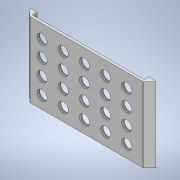
# Autodesk Inventor part: PalmSupport
Saved by Autodesk Inventor 2020 (Build 240168000, 168)
## iProperties
Created: 2019-10-21
Part Number: PalmSupport
Material: Generic
Document SubType Name: Modeling
Designer: ayad493
Density: 1 g/cm^3
Appearance: Default
Author: ayad493
Autodesk Inventor part; units mm, degrees
ref_plane "YZ Plane" through (0, 0, 0) normal (1, 0, 0) x (0, 1, 0)
ref_plane "XZ Plane" through (0, 0, 0) normal (0, 1, 0) x (-1, 0, 0)
ref_plane "XY Plane" through (0, 0, 0) normal (0, 0, 1) x (1, 0, 0)
sketch "Sketch1" plane through (0, 0, 0) normal (0, 0, 1) x (1, 0, 0)
  line L0 (0, 0) -> (51.5, 0)
  line L1 (51.5, 0) -> (51.5, 30)
  line L2 (51.5, 30) -> (0, 30)
  line L3 (0, 30) -> (0, 0)
  dimension "d0" = 51.5
  dimension "d1" = 30
  constraints: 8 end point, 2 parallel, 1 horizontal, 1 perpendicular
  measures "d0" distance of L2.end L1.end
  measures "d1" distance of L1.end L0.end
extrude "Extrusion1" add sketch "Sketch1" along normal blind 2.9
sketch "Sketch2" plane through (0, 0, 0) normal (0, -1, 0) x (1, 0, 0)
  line L0 (0, 0) -> (0, 2.9) projected
  line L1 (0, 2.9) -> (3, 2.9)
  line L2 (51.5, 2.9) -> (0, 2.9) projected
  line L3 (51.5, 0) -> (0, 0) projected
  line L4 (3, 2.9) -> (0, 0)
  line L5 (51.5, 2.9) -> (48.5, 2.9)
  line L6 (48.5, 2.9) -> (51.5, 0)
  line L7 (3, 2.9) -> (3, 0)
  line L8 (3, 0) -> (48, 0)
  line L9 (48, 0) -> (48, 1.9)
  line L10 (48, 1.9) -> (3, 1.9)
  line L11 (3, 1.9) -> (3, 0)
  line L12 (51.5, 2.9) -> (51.5, 0)
  dimension "d4" = 3
  dimension "d5" = 3
  dimension "d6" = 1.9
  constraints: 20 end point, 4 point on line, 3 perpendicular, 2 parallel, 1 horizontal
  measures "d4" distance of L0.end L1.end
  measures "d5" distance of L2.start L5.end
  measures "d6" distance of L9.end L8.end
extrude "Extrusion2" cut sketch "Sketch2" against normal through all contours L0 L1 L4 | L7 L10 L9 L3 | L2 L12 L6
fillet "Fillet1" radius 0.3 4 edges at (3, 15, 2.9) (0, 15, 0) (48.5, 15, 2.9) (51.5, 15, 0)
sketch "Sketch4" plane through (48, 0, 1.9) normal (0, 0, -1) x (-1, 0, 0)
  line L0 (45, 0) -> (0, 0) projected
  line L1 (45, 0) -> (40, 0)
  line L2 (40, 0) -> (40, 5)
  circle A0 centre (40, 5) radius 2
  circle A1 centre (31.5, 5) radius 2
  circle A2 centre (23, 5) radius 2
  circle A3 centre (14.5, 5) radius 2
  circle A4 centre (6, 5) radius 2
  circle A5 centre (40, 11.5) radius 2
  circle A6 centre (31.5, 11.5) radius 2
  circle A7 centre (23, 11.5) radius 2
  circle A8 centre (14.5, 11.5) radius 2
  circle A9 centre (6, 11.5) radius 2
  circle A10 centre (40, 18) radius 2
  circle A11 centre (31.5, 18) radius 2
  circle A12 centre (23, 18) radius 2
  circle A13 centre (14.5, 18) radius 2
  circle A14 centre (6, 18) radius 2
  circle A15 centre (40, 24.5) radius 2
  circle A16 centre (31.5, 24.5) radius 2
  circle A17 centre (23, 24.5) radius 2
  circle A18 centre (14.5, 24.5) radius 2
  circle A19 centre (6, 24.5) radius 2
  point P0 (48, 0)
  dimension "d10" = 5
  dimension "d11" = 5
  dimension "d12" = 4
  dimension "d15" = 8.5
  dimension "d18" = 6.5
  constraints: 20 centre point, 4 end point, 1 coincident, 1 horizontal, 1 perpendicular, 1 point on line, 1 vertical, 38 other
  measures "d10" distance of L0.start L1.end
  measures "d11" distance of L1.end L2.end
  measures "d12" diameter of A0
  measures "d15" distance of A0.centre A1.centre
  measures "d18" distance of A0.centre A5.centre
extrude "Extrusion3" cut sketch "Sketch4" against normal blind 2.9
body "Solid1"
